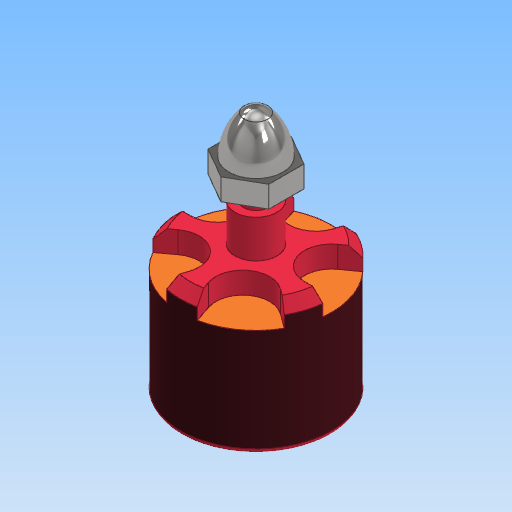
# Autodesk Inventor part: Моторчик
Saved by Autodesk Inventor 2021.2 (Build 252289000, 289)
## iProperties
Created: 2024-10-29
Part Number: Моторчик
Material: Типовые
Document SubType Name: Modeling
Designer: barko
Density: 3.38458 g/cm^3
Appearance: Сталь — полированная
Mass: 50 g
Surface Area: 42.6412 cm^2
Volume: 14.7729 cm^3
Author: barko
Autodesk Inventor part; units mm, degrees
ref_plane "YZ Plane" through (0, 0, 0) normal (1, 0, 0) x (0, 1, 0)
ref_plane "XZ Plane" through (0, 0, 0) normal (0, 1, 0) x (-1, 0, 0)
ref_plane "XY Plane" through (0, 0, 0) normal (0, 0, 1) x (1, 0, 0)
sketch "Эскиз1" plane through (0, 0, 0) normal (0, 0, 1) x (1, 0, 0)
  line L0 (0, 0) -> (0, 31)
  line L1 (0, 0) -> (-14, 0)
  line L2 (-14, 0) -> (-14, 24)
  line L3 (-14, 24) -> (-3.9, 24)
  line L4 (-3.9, 24) -> (-3.9, 31)
  line L5 (-3.9, 31) -> (0, 31)
  line L6 (-3.05, 0) -> (-3.05, -1.9)
  line L7 (-3.05, -1.9) -> (0, -1.9)
  line L8 (0, -1.9) -> (0, 0)
  line L9 (0, 38) -> (0, 31)
  line L10 (-2.35, 31) -> (-2.35, 32.5)
  line L11 (-2.35, 32.5) -> (-3, 32.5)
  line L12 (-3, 32.5) -> (-3, 38)
  line L13 (-3, 38) -> (0, 38)
  dimension "d0" = 24
  dimension "d1" = 28
  dimension "d2" = 7.8
  dimension "d3" = 7
  dimension "d5" = 6.1
  dimension "d6" = 1.9
  dimension "d20" = 4.7
  dimension "d21" = 6
  dimension "d22" = 7
  dimension "d23" = 1.5
  constraints: 29 end point, 7 perpendicular, 4 vertical, 2 point on line, 1 horizontal, 1 parallel, 1 vertical alignment
  measures "d0" distance between parallel lines of L3 L1
  measures "d1" diameter of L2 L0
  measures "d2" diameter of L4 L0
  measures "d3" distance between parallel lines of L3 L5
  measures "d5" diameter of L6 L0
  measures "d6" distance between parallel lines of L1 L7
  measures "d20" diameter of L10 L9
  measures "d21" diameter of L12 L9
  measures "d22" distance between parallel lines of L5 L13
  measures "d23" distance of L10.start L10.end
revolve "Вращение1" add sketch "Эскиз1" angle 360 about axis through (0, 0, 0) along (0, 1, 0)
chamfer "Фаска1" distance 1.8526 angle 45 1 edges at (14, 24, 0)
fillet "Сопряжение1" radius 1 1 edges at (14, 0, 0)
sketch "Эскиз2" plane through (0, 24, 0) normal (0, 1, 0) x (1, 0, 0)
  line L0 (-5.7653, 12.7578) -> (-4.7686, 9.5965)
  arc A0 (-4.7686, 9.5965) -> (4.7686, 9.5965) centre (0, 11.1) ccw
  line L1 (4.7686, 9.5965) -> (5.7653, 12.7578)
  circle A1 centre (0, 0) radius 14 projected
  point P0 (0, 0)
  dimension "d11" = 7.9
  dimension "d12" = 35
  dimension "d13" = 5
  constraints: 4 end point, 4 point on circle, 2 tangent, 1 centre point, 1 equal length, 1 vertical alignment
  measures "d12" angle of L1 L0
  measures "d13" radius of A0
extrude "Выдавливание1" cut sketch "Эскиз2" against normal blind 4 contours A1 L1 A0 L0 picked at (2.4163, 12.0782)
pattern_circular "Круговой массив1" count 5 over 360 about axis through (0, 12, 0) along (0, 1, 0) of "Выдавливание1"
thread "Резьба1" size "M6x1" class "6g" standard "ISO Metric profile" full length
chamfer "Фаска2" distance 0.5 angle 45 1 edges at (3, 38, 0)
sketch "Эскиз4" plane through (0, 0, 0) normal (0, 0, 1) x (1, 0, 0)
  line L0 (0, 34) -> (-6.5, 34)
  line L1 (-6.5, 34) -> (-6.5, 38)
  line L2 (-6.5, 38) -> (-5, 38)
  arc A0 (-2.1724, 45.069) -> (-5, 38) centre (5.25, 38) ccw
  line L3 (0, 34) -> (0, 46)
  arc A1 (0, 46) -> (-2.1724, 45.069) centre (0, 43) ccw
  point P0 (0, 0)
  dimension "d8" = 2
  dimension "d52" = 4
  dimension "d53" = 10
  dimension "d54" = 3
  dimension "d55" = 13
  dimension "d60" = 12
  constraints: 8 end point, 4 point on circle, 2 centre point, 2 perpendicular, 1 horizontal, 1 line through centre, 1 point on line, 1 tangent, 1 vertical, 1 vertical alignment
  measures "d52" distance of L0.end L1.end
  measures "d53" diameter of L2.end L3
  measures "d54" radius of A1
  measures "d55" diameter of L1 L3
  measures "d60" distance of L0.start L3.end
revolve "Вращение3" add sketch "Эскиз4" angle 360 about axis through (0, 34, 0) along (0, 1, 0) separate body
sketch "Эскиз5" plane through (0, 38, 0) normal (0, 1, 0) x (1, 0, 0)
  circle A0 centre (0, 0) radius 6.5 projected
  circle A1 centre (0, 0) radius 3.05 construction
  line L0 (0, 6.5) -> (5.6292, 3.25)
  line L1 (5.6292, 3.25) -> (5.6292, -3.25)
  line L2 (5.6292, -3.25) -> (0, -6.5)
  line L3 (0, -6.5) -> (-5.6292, -3.25)
  line L4 (-5.6292, -3.25) -> (-5.6292, 3.25)
  line L5 (-5.6292, 3.25) -> (0, 6.5)
  point P0 (-5.6292, 3.25)
  point P1 (-5.6292, 3.25)
  point P2 (-5.6292, -3.25)
  point P3 (-5.6292, -3.25)
  point P4 (0, -6.5)
  point P5 (0, -6.5)
  point P6 (5.6292, -3.25)
  point P7 (5.6292, -3.25)
  point P8 (5.6292, 3.25)
  point P9 (5.6292, 3.25)
  constraints: 12 end point, 1 coincident, 1 vertical, 15 other
extrude "Выдавливание3" cut sketch "Эскиз5" against normal up to surface (4 mm away) contours A0 L1 | L0 A0 | A0 L2 | L5 A0 | A0 L3 | L4 A0 bodies 2
equation "\"d0\" = motor_height"
equation "\"d1\" = motor_diameter"
equation "\"blade_radius\" = 127"
equation "\"bearing_inner\" = 7"
equation "\"bearing_outer\" = 19"
equation "\"bearing_width\" = 6"
equation "\"beam_length\" = 254"
equation "\"motor_height\" = 24"
equation "\"motor_diameter\" = 28"
equation "\"motor_blade_offset\" = 2"
equation "\"M4_nut_lock_width\" = 6.8"
equation "\"M4_screw_innerHex_cap_diam\" = 6.6"
equation "\"M4_screw_innerHex_cap_height\" = 4"
equation "\"M4_nut_lock_height\" = 5"
